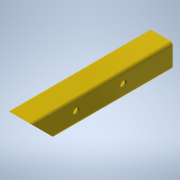
# Autodesk Inventor part: beam 25x25x2 2-2
Saved by Autodesk Inventor 2021 (Build 250183000, 183)
## iProperties
Created: 2024-04-08
Part Number: beam 25x25x2 2-2
Material: Steel
Document SubType Name: Modeling
Designer: Michal
Density: 7.85 g/cm^3
Appearance: Glossy - Gold
Author: Michal
Autodesk Inventor part; units mm, degrees
ref_plane "YZ Plane" through (0, 0, 0) normal (1, 0, 0) x (0, 1, 0)
ref_plane "XZ Plane" through (0, 0, 0) normal (0, 1, 0) x (-1, 0, 0)
ref_plane "XY Plane" through (0, 0, 0) normal (0, 0, 1) x (1, 0, 0)
sketch "Sketch1" plane through (0, 0, 0) normal (0, 1, 0) x (-1, 0, 0)
  line L0 (-9.5, 11.5) -> (9.5, 11.5) construction
  line L1 (11.5, 9.5) -> (11.5, -9.5) construction
  line L2 (9.5, -11.5) -> (-9.5, -11.5) construction
  line L3 (-11.5, -9.5) -> (-11.5, 9.5) construction
  line L4 (-11.5, 11.5) -> (11.5, -11.5) construction
  line L5 (11.5, 11.5) -> (-11.5, -11.5) construction
  arc A0 (11.5, 9.5) -> (9.5, 11.5) centre (9.5, 9.5) ccw construction
  arc A1 (9.5, -11.5) -> (11.5, -9.5) centre (9.5, -9.5) ccw construction
  arc A2 (-11.5, -9.5) -> (-9.5, -11.5) centre (-9.5, -9.5) ccw construction
  arc A3 (-9.5, 11.5) -> (-11.5, 9.5) centre (-9.5, 9.5) ccw construction
  line L6 (-9.5, -12.5) -> (9.5, -12.5)
  arc A4 (9.5, -12.5) -> (12.5, -9.5) centre (9.5, -9.5) ccw
  line L7 (12.5, -9.5) -> (12.5, 9.5)
  arc A5 (12.5, 9.5) -> (9.5, 12.5) centre (9.5, 9.5) ccw
  line L8 (9.5, 12.5) -> (-9.5, 12.5)
  arc A6 (-9.5, 12.5) -> (-12.5, 9.5) centre (-9.5, 9.5) ccw
  line L9 (-12.5, 9.5) -> (-12.5, -9.5)
  arc A7 (-12.5, -9.5) -> (-9.5, -12.5) centre (-9.5, -9.5) ccw
  line L10 (10.5, -9.5) -> (10.5, 9.5)
  arc A8 (10.5, 9.5) -> (9.5, 10.5) centre (9.5, 9.5) ccw
  line L11 (9.5, 10.5) -> (-9.5, 10.5)
  arc A9 (-9.5, 10.5) -> (-10.5, 9.5) centre (-9.5, 9.5) ccw
  line L12 (-10.5, 9.5) -> (-10.5, -9.5)
  arc A10 (-10.5, -9.5) -> (-9.5, -10.5) centre (-9.5, -9.5) ccw
  line L13 (-9.5, -10.5) -> (9.5, -10.5)
  arc A11 (9.5, -10.5) -> (10.5, -9.5) centre (9.5, -9.5) ccw
  point P0 (0, 0)
  point P1 (0, 0)
  point P2 (0, 0)
  dimension "d10" = 2
  dimension "depth" = 25
  dimension "width" = 25
  dimension "thickness" = 2
  constraints: 28 end point, 24 point on circle, 12 centre point, 8 point on line, 8 tangent, 6 parallel, 3 equal radius, 3 midpoint, 3 perpendicular, 1 coincident, 1 horizontal, 15 other
  measures "d10" radius of A0
  measures "depth" distance between parallel lines of L6 L8
  measures "width" distance between parallel lines of L9 L7
  measures "thickness" distance between parallel lines of L10 L7
extrude "Extrusion1" add sketch "Sketch1" along normal blind 150
sketch "Sketch2" plane through (12.5, 0, 9.5) normal (1, 0, 0) x (0, 0, -1)
  line L0 (9.5, -30) -> (9.5, 180) construction
  line L1 (0, 150) -> (19, 150) projected
  point P0 (9.5, 0)
  point P1 (9.5, 98)
  point P2 (9.5, 48)
  dimension "d16" = 52
  dimension "d17" = 50
  constraints: 2 point on line
  measures "d16" distance from line of point (9.5, 98) L1
  measures "d17" distance of point (9.5, 48) point (9.5, 98)
hole "Hole1" at (12.5, 98, 0) at (12.5, 48, 0) direction (-1, 0, 0) diameter 6.647 depth 20.2 tip angle 118 thread size "M8x1.25" class "6H" standard "ANSI Metric M Profile"
draft "FaceDraft2" angle -45 pull direction (0, 0, 1) fixed plane through (3.1667, 50, 12.5) normal (0, 0, 1) faces at (3.1667, 0, -11.8333)
equation "\"d10\" = thickness"
body "Solid1"
